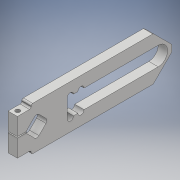
# Autodesk Inventor part: came
Saved by Autodesk Inventor 2017 (Build 210142000, 142)
## iProperties
Part Number: came
Material: Générique
Document SubType Name: Modeling
Designer: allais
Density: 1 g/cm^3
Appearance: Par défaut
Author: allais
Autodesk Inventor part; units mm, degrees
ref_plane "YZ Plane" through (0, 0, 0) normal (1, 0, 0) x (0, 1, 0)
ref_plane "XZ Plane" through (0, 0, 0) normal (0, 1, 0) x (-1, 0, 0)
ref_plane "XY Plane" through (0, 0, 0) normal (0, 0, 1) x (1, 0, 0)
sketch "Esquisse1" plane through (0, 0, 0) normal (1, 0, 0) x (0, 1, 0)
  line L0 (0, 0) -> (122.5, 0)
  line L1 (217, 0) -> (217, 4.1716)
  line L2 (216.4142, 5.5858) -> (187.5858, 34.4142)
  line L3 (186.1716, 35) -> (-6.5, 35)
  line L4 (-9, 32.5) -> (-9, 31.5)
  line L5 (-11.5, 29) -> (-31, 29)
  line L6 (-31, 29) -> (-31, 1)
  line L7 (-31, 1) -> (0, 1)
  line L8 (0, 1) -> (0, 0)
  arc A0 (217, 4.1716) -> (216.4142, 5.5858) centre (215, 4.1716) ccw
  arc A1 (187.5858, 34.4142) -> (186.1716, 35) centre (186.1716, 33) ccw
  arc A2 (-6.5, 35) -> (-9, 32.5) centre (-6.5, 32.5) ccw
  arc A3 (-11.5, 29) -> (-9, 31.5) centre (-11.5, 31.5) ccw
  line L9 (217, 0) -> (217, -4.1716)
  line L10 (216.4142, -5.5858) -> (187.5858, -34.4142)
  line L11 (186.1716, -35) -> (-6.5, -35)
  line L12 (-9, -32.5) -> (-9, -31.5)
  line L13 (-11.5, -29) -> (-31, -29)
  line L14 (-31, -29) -> (-31, -1)
  line L15 (-31, -1) -> (0, -1)
  line L16 (0, -1) -> (0, 0)
  arc A4 (216.4142, -5.5858) -> (217, -4.1716) centre (215, -4.1716) ccw
  arc A5 (186.1716, -35) -> (187.5858, -34.4142) centre (186.1716, -33) ccw
  arc A6 (-9, -32.5) -> (-6.5, -35) centre (-6.5, -32.5) ccw
  arc A7 (-9, -31.5) -> (-11.5, -29) centre (-11.5, -31.5) ccw
  point P0 (217, 5)
  point P1 (217, -5)
  dimension "d0" = 70
  dimension "d1" = 10
  dimension "d2" = 45
  dimension "d3" = 31
  dimension "d4" = 22
  dimension "d5" = 217
  dimension "d6" = 58
  dimension "d7" = 2
  dimension "d8" = 2
  dimension "d9" = 2.5
  constraints: 34 end point, 16 point on circle, 16 symmetric about line, 8 centre point, 8 tangent, 6 perpendicular, 5 point on line, 2 equal radius, 1 horizontal, 1 vertical, 4 other
  measures "d0" diameter of L3 L0
  measures "d1" diameter of point (217, 5) L0
  measures "d2" angle of L3 L2
  measures "d3" distance from line of L0.start L6
  measures "d4" distance between parallel lines of L6 L4
  measures "d5" distance between parallel lines of L8 L1
  measures "d6" diameter of L5 L0
  measures "d7" diameter of L7 L0
  measures "d8" radius of A0
  measures "d9" radius of A2
extrude "Extrusion1" add sketch "Esquisse1" along normal blind 15
sketch "Esquisse2" plane through (15, 0, 0) normal (1, 0, 0) x (0, 0, -1)
  line L0 (0, 210) -> (0, 210)
  line L1 (15, 49) -> (-15, 49)
  line L2 (4.1716, 217) -> (-4.1716, 217) projected
  arc A0 (0, 210) -> (-15, 195) centre (0, 195) ccw
  arc A1 (15, 195) -> (0, 210) centre (0, 195) ccw
  line L3 (1, -31) -> (29, -31) projected
  line L4 (-3.5355, 14.8492) -> (-14.8492, 3.5355)
  line L5 (-14.8492, -3.5355) -> (-3.5355, -14.8492)
  line L6 (3.5355, -14.8492) -> (14.8492, -3.5355)
  line L7 (14.8492, 3.5355) -> (3.5355, 14.8492)
  arc A2 (3.5355, 14.8492) -> (-3.5355, 14.8492) centre (0, 11.3137) ccw
  arc A3 (14.8492, -3.5355) -> (14.8492, 3.5355) centre (11.3137, 0) ccw
  arc A4 (-3.5355, -14.8492) -> (3.5355, -14.8492) centre (0, -11.3137) ccw
  arc A5 (-14.8492, 3.5355) -> (-14.8492, -3.5355) centre (-11.3137, 0) ccw
  line L8 (-35, 186.1716) -> (-35, -6.5) projected
  line L9 (-1, 0) -> (1, 0) projected
  arc A6 (15, 49) -> (15, 59) centre (15, 54) ccw
  arc A7 (-15, 59) -> (-15, 49) centre (-15, 54) ccw
  arc A8 (-15, 76) -> (-15, 66) centre (-15, 71) ccw
  line L10 (-15, 59) -> (-15, 66)
  line L11 (-15, 76) -> (-15, 195)
  arc A9 (15, 66) -> (15, 76) centre (15, 71) ccw
  line L12 (15, 195) -> (15, 76)
  line L13 (15, 66) -> (15, 59)
  point P0 (0, 0)
  point P1 (-15, 210)
  point P2 (15, 210)
  point P3 (0, 18.3848)
  point P4 (-18.3848, 0)
  point P5 (18.3848, 0)
  point P6 (0, 0)
  point P7 (0, 0)
  dimension "d12" = 30
  dimension "d14" = 7
  dimension "d15" = 15
  dimension "d16" = 80
  dimension "d17" = 26
  dimension "d18" = 26
  dimension "d19" = 5
  dimension "d20" = 45
  dimension "d21" = 10
  dimension "d22" = 10
  dimension "d23" = 10
  dimension "d24" = 12
  dimension "d25" = 10
  dimension "d26" = 30
  dimension "d27" = 15
  constraints: 20 end point, 20 point on circle, 16 tangent, 10 centre point, 8 point on line, 5 parallel, 5 perpendicular, 4 equal radius, 2 horizontal alignment, 2 midpoint, 1 horizontal, 1 vertical alignment
  measures "d12" distance of point (-15, 210) point (15, 210)
  measures "d14" distance between parallel lines of L2 L0
  measures "d15" radius of A0
  measures "d16" distance between parallel lines of L3 L1
  measures "d17" distance of point (0, 18.385) point (-18.385, 0)
  measures "d18" distance of point (18.385, 0) point (0, 18.385)
  measures "d19" radius of A2
  measures "d20" angle of L8 L5
  measures "d21" diameter of A6
  measures "d22" diameter of A7
  measures "d23" diameter of A8
  measures "d24" distance of L10.start A8.centre
  measures "d25" diameter of A9
  measures "d26" distance between parallel lines of L12 L11
  measures "d27" distance from line of point (0, 0) L11
extrude "Extrusion2" cut sketch "Esquisse2" against normal through all
sketch "Esquisse3" plane through (0, -31, 29) normal (0, 0, 1) x (1, 0, 0)
  line L0 (0, 0) -> (0, 19.5) projected
  line L1 (0, 0) -> (15, 0) projected
  point P0 (0, 31)
  point P1 (7.5, 8)
  dimension "d30" = 7.5
  dimension "d31" = 8
  measures "d30" distance from line of L0 point (7.5, 8)
  measures "d31" distance from line of L1 point (7.5, 8)
hole "Perçage1" at (7.5, -23, 29) direction (0, 0, -1) diameter 7 end through all
